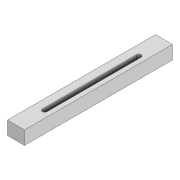
# Autodesk Inventor part: Rail
Saved by Autodesk Inventor 2022 (Build 260153000, 153)
## iProperties
Created: 2022-04-23
Part Number: Rail
Material: Generic
Document SubType Name: Modeling
Designer: dell
Density: 1 g/cm^3
Appearance: Default
Author: dell
Autodesk Inventor part; units mm, degrees
ref_plane "YZ Plane" through (0, 0, 0) normal (1, 0, 0) x (0, 1, 0)
ref_plane "XZ Plane" through (0, 0, 0) normal (0, 1, 0) x (-1, 0, 0)
ref_plane "XY Plane" through (0, 0, 0) normal (0, 0, 1) x (1, 0, 0)
sketch "Sketch1" plane through (0, 0, 0) normal (0, 1, 0) x (-1, 0, 0)
  line L0 (0, 0) -> (0, -70) construction
  line L1 (-1.65, 0) -> (-1.65, -70)
  line L2 (1.65, -70) -> (1.65, 0)
  arc A0 (1.65, 0) -> (-1.65, 0) centre (0, 0) ccw
  arc A1 (-1.65, -70) -> (1.65, -70) centre (0, -70) ccw
  line L3 (-5, 20) -> (7.65, 20)
  line L4 (7.65, 20) -> (7.65, -90)
  line L5 (7.65, -90) -> (-5, -90)
  line L6 (-5, -90) -> (-5, 20)
  circle A2 centre (0, -70) radius 5
  circle A3 centre (0, 0) radius 5
  point P0 (0, -35)
  dimension "d0" = 3.3
  dimension "d1" = 70
  dimension "d2" = 10
  dimension "d3" = 10
  dimension "d4" = 20
  dimension "d5" = 20
  dimension "d6" = 6
  constraints: 16 end point, 5 tangent, 4 centre point, 4 point on circle, 3 parallel, 2 coincident, 1 horizontal, 1 midpoint, 1 perpendicular, 1 vertical
  measures "d0" diameter of A1
  measures "d1" distance of L0.start L0.end
  measures "d2" diameter of A2
  measures "d3" diameter of A3
  measures "d4" distance from line of L0.start L3
  measures "d5" distance from line of L5 L0.end
  measures "d6" distance between parallel lines of L4 L2
extrude "Extrusion1" add sketch "Sketch1" along normal blind 10 contours L1 A3 L2 A0 | L1 A2 L6 A3 | L1 A1 L2 A2 | L6 L3 L4 L5 A2 L2 A3 picked at (-2.0178, -2.9645) picked at (-2.0178, -67.0355)
body "Solid1"
